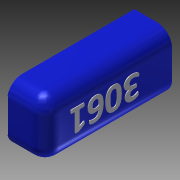
# Autodesk Inventor part: Bumper Cover Part4 (26x28 robot)
Saved by Autodesk Inventor 2014 SP1 (Build 180222100, 222)
## iProperties
Created: 2013-01-06
Part Number: Bumper Cover Part4 (26x28 robot)
Material: Generic
Document SubType Name: Modeling
Designer: Moses
Density: 1 g/cm^3
Mass: 183.688 g
Surface Area: 2193.04 cm^2
Volume: 183.688 cm^3
Appearance: Blue - Wall Paint - Glossy
Author: Moses
Autodesk Inventor part; units mm, degrees
ref_plane "YZ Plane" through (0, 0, 0) normal (1, 0, 0) x (0, 1, 0)
ref_plane "XZ Plane" through (0, 0, 0) normal (0, 1, 0) x (-1, 0, 0)
ref_plane "XY Plane" through (0, 0, 0) normal (0, 0, 1) x (1, 0, 0)
sketch "Sketch1" plane through (0, 0, 0) normal (0, 0, 1) x (1, 0, 0)
  circle A0 centre (38.1, -31.75) radius 31.75 construction
  circle A1 centre (38.1, 31.75) radius 31.75 construction
  line L0 (6.35, 63.5) -> (38.1, 63.5) construction
  line L1 (69.85, 31.75) -> (69.85, -31.75) construction
  line L2 (6.35, -63.5) -> (38.1, -63.5) construction
  line L3 (38.1, 65.0875) -> (-14.2875, 65.0875)
  line L4 (-14.2875, -65.0875) -> (38.1, -65.0875)
  arc A2 (38.1, -65.0875) -> (71.4375, -31.75) centre (38.1, -31.75) ccw
  arc A3 (71.4375, 31.75) -> (38.1, 65.0875) centre (38.1, 31.75) ccw
  line L5 (71.4375, 31.75) -> (71.4375, -31.75)
  line L6 (38.1, 65.0875) -> (38.1, 63.5) construction
  arc A4 (69.85, 31.75) -> (38.1, 63.5) centre (38.1, 31.75) ccw
  arc A5 (38.1, -63.5) -> (69.85, -31.75) centre (38.1, -31.75) ccw
  line L7 (69.85, 31.75) -> (69.85, -31.75)
  line L8 (-12.7, 63.5) -> (-12.7, 38.1)
  line L9 (-12.7, 38.1) -> (-14.2875, 38.1)
  line L10 (-14.2875, 38.1) -> (-14.2875, 65.0875)
  line L11 (-14.2875, -65.0875) -> (-14.2875, -38.1)
  line L12 (-14.2875, -38.1) -> (-12.7, -38.1)
  line L13 (-12.7, -63.5) -> (-12.7, -38.1)
  line L14 (-12.7, 38.1) -> (-12.7, -38.1)
  line L15 (-12.7, -63.5) -> (-12.7, 63.5) construction
  line L16 (-12.7, 63.5) -> (6.35, 63.5) construction
  line L17 (6.35, 63.5) -> (6.35, -63.5) construction
  line L18 (6.35, -63.5) -> (-12.7, -63.5) construction
  line L19 (-12.7, 63.5) -> (38.1, 63.5)
  line L20 (-12.7, -63.5) -> (38.1, -63.5)
  point P0 (0, 0)
  point P1 (38.1, 64.2937)
  dimension "d3" = 25.4
  dimension "d7" = 25.4
  dimension "d9" = 1.5875
  dimension "d20" = 1.5875
  dimension "d21" = 1.5875
  constraints: 34 end point, 14 tangent, 12 point on circle, 5 parallel, 4 centre point, 4 perpendicular, 2 coincident, 2 point on line, 1 collinear, 1 concentric, 1 midpoint, 1 vertical
  measures "d3" distance of L8.start L8.end
  measures "d7" distance of L13.start L12.end
  measures "d9" distance of L3.start L0.end
  measures "d20" distance of L11.end L12.end
  measures "d21" distance of L8.end L9.end
extrude "Extrusion1" add sketch "Sketch1" along normal blind 1.5875
extrude "Extrusion2" add sketch "Sketch1" against normal blind 285.75 contours A3 L5 A2 L4 L11 L12 L13 L20 A5 L7 A4 L19 L8 L9 L10 L3
sketch "Sketch2" plane through (0, 0, -285.75) normal (0, 0, -1) x (-1, 0, 0)
  arc A0 (-38.1, 63.5) -> (-69.85, 31.75) centre (-38.1, 31.75) ccw projected
  line L0 (-38.1, 63.5) -> (12.7, 63.5) projected
  line L1 (12.7, 63.5) -> (12.7, 38.1) projected
  line L2 (12.7, 38.1) -> (14.2875, 38.1) projected
  line L3 (14.2875, 38.1) -> (14.2875, 65.0875) projected
  line L4 (14.2875, 65.0875) -> (-38.1, 65.0875) projected
  arc A1 (-38.1, 65.0875) -> (-71.4375, 31.75) centre (-38.1, 31.75) ccw projected
  line L5 (-71.4375, 31.75) -> (-71.4375, -31.75) projected
  arc A2 (-71.4375, -31.75) -> (-38.1, -65.0875) centre (-38.1, -31.75) ccw projected
  line L6 (-38.1, -65.0875) -> (14.2875, -65.0875) projected
  line L7 (14.2875, -65.0875) -> (14.2875, -38.1) projected
  line L8 (14.2875, -38.1) -> (12.7, -38.1) projected
  line L9 (12.7, -38.1) -> (12.7, -63.5) projected
  line L10 (12.7, -63.5) -> (-38.1, -63.5) projected
  arc A3 (-69.85, -31.75) -> (-38.1, -63.5) centre (-38.1, -31.75) ccw projected
  line L11 (-69.85, -31.75) -> (-69.85, 31.75) projected
  line L12 (12.7, -63.5) -> (12.7, 63.5) projected
extrude "Extrusion3" add sketch "Sketch2" along normal blind 1.5875
fillet "Fillet1" radius 33.3375 8 edges at (61.6732, -55.3232, 1.5875) (71.4375, 0, 1.5875) (61.6732, 55.3232, 1.5875) (11.9063, 65.0875, 1.5875) (11.9062, -65.0875, 1.5875) (60.5506, -54.2006, 0) (69.85, 0, 0) (60.5506, 54.2006, 0)
sketch "Sketch3" plane through (71.4375, -31.75, -287.3375) normal (1, 0, 0) x (0, 0, -1)
  line L0 (-255.5875, 0) -> (-255.5875, 63.5) projected
  line L1 (0, 0) -> (-255.5875, 0) projected
  line L2 (0, 63.5) -> (-255.5875, 63.5) projected
  line L3 (-77.7875, 0) -> (-230.1875, 0) construction
  line L4 (-230.1875, 0) -> (-230.1875, 63.5) construction
  line L5 (-230.1875, 63.5) -> (-77.7875, 63.5) construction
  line L6 (-77.7875, 63.5) -> (-77.7875, 0) construction
  spline S0 degree 2 poles (-110.0562, 42.2439) (-110.0562, 46.0122) (-107.1466, 51.8792) (-101.995, 55.886) (-94.7924, 57.937) (-90.5471, 57.937) knots 0 0 0 1 2 3 4 4 4
  spline S1 degree 2 poles (-90.5471, 57.937) (-87.9714, 57.937) (-83.4399, 57.1738) (-79.9578, 56.1245) (-77.6683, 54.932) (-77.0005, 54.3119) (-76.6189, 53.501) (-76.3327, 52.4516) (-76.2373, 50.8775) (-76.2373, 49.7327) knots 0 0 0 1 2 3 4 5 6 7 8 8 8
  spline S2 degree 2 poles (-76.2373, 49.7327) (-76.2373, 47.8247) (-76.8574, 46.3938) (-77.4775, 46.3938) knots 0 0 0 1 2 2 2
  spline S3 degree 2 poles (-77.4775, 46.3938) (-77.8591, 46.3938) (-79.8147, 47.4431) (-82.7721, 48.6833) (-86.7789, 49.7327) (-89.3069, 49.7327) knots 0 0 0 1 2 3 4 4 4
  spline S4 degree 2 poles (-89.3069, 49.7327) (-91.4534, 49.7327) (-94.7447, 48.731) (-97.0343, 46.8707) (-98.179, 44.2473) (-98.179, 42.6732) knots 0 0 0 1 2 3 4 4 4
  spline S5 degree 2 poles (-98.179, 42.6732) (-98.179, 40.9083) (-96.7958, 38.094) (-94.1246, 36.0907) (-90.0224, 34.9936) (-87.2082, 34.9936) knots 0 0 0 1 2 3 4 4 4
  line L7 (-87.2082, 34.9936) -> (-82.8198, 34.9936)
  spline S6 degree 2 poles (-82.8198, 34.9936) (-82.3428, 34.9936) (-81.6273, 34.7074) (-81.1503, 33.8488) (-80.9595, 32.3224) (-80.9595, 31.1299) knots 0 0 0 1 2 3 4 4 4
  spline S7 degree 2 poles (-80.9595, 31.1299) (-80.9595, 29.9851) (-81.1503, 28.5541) (-81.5796, 27.7909) (-82.2474, 27.457) (-82.7244, 27.457) knots 0 0 0 1 2 3 4 4 4
  line L8 (-82.7244, 27.457) -> (-87.1605, 27.457)
  spline S8 degree 2 poles (-87.1605, 27.457) (-89.45, 27.457) (-92.9798, 26.4077) (-95.3648, 24.452) (-96.605, 21.6854) (-96.605, 19.9682) knots 0 0 0 1 2 3 4 4 4
  spline S9 degree 2 poles (-96.605, 19.9682) (-96.605, 18.6803) (-95.7464, 16.3908) (-94.0769, 14.7213) (-91.4057, 13.7196) (-89.5931, 13.7196) knots 0 0 0 1 2 3 4 4 4
  spline S10 degree 2 poles (-89.5931, 13.7196) (-87.5421, 13.7196) (-83.9646, 14.9121) (-81.1026, 16.3908) (-79.0992, 17.6309) (-78.6222, 17.6309) knots 0 0 0 1 2 3 4 4 4
  spline S11 degree 2 poles (-78.6222, 17.6309) (-78.336, 17.6309) (-77.8591, 17.3447) (-77.5252, 16.5815) (-77.3821, 15.1029) (-77.3821, 13.9104) knots 0 0 0 1 2 3 4 4 4
  spline S12 degree 2 poles (-77.3821, 13.9104) (-77.3821, 12.9564) (-77.4775, 11.6685) (-77.716, 10.8099) (-78.0498, 10.1898) (-78.813, 9.4266) (-81.2457, 7.9479) (-84.9186, 6.5169) (-89.7362, 5.563) (-92.5505, 5.563) knots 0 0 0 1 2 3 4 5 6 7 8 8 8
  spline S13 degree 2 poles (-92.5505, 5.563) (-96.2234, 5.563) (-101.8996, 7.2801) (-105.7633, 10.5237) (-107.7667, 15.246) (-107.7667, 18.251) knots 0 0 0 1 2 3 4 4 4
  spline S14 degree 2 poles (-107.7667, 18.251) (-107.7667, 20.5406) (-106.5742, 24.4997) (-104.3323, 27.6478) (-100.8979, 29.842) (-98.7037, 30.3667) knots 0 0 0 1 2 3 4 4 4
  line L9 (-98.7037, 30.3667) -> (-98.7037, 30.5098)
  spline S15 degree 2 poles (-98.7037, 30.5098) (-101.3272, 30.796) (-105.5725, 32.8948) (-108.4821, 35.9953) (-110.0562, 39.9543) (-110.0562, 42.2439) knots 0 0 0 1 2 3 4 4 4
  spline S16 degree 2 poles (-151.841, 31.5592) (-151.841, 37.617) (-149.8853, 47.3954) (-145.4493, 54.2642) (-138.3898, 57.937) (-133.2859, 57.937) knots 0 0 0 1 2 3 4 4 4
  spline S17 degree 2 poles (-133.2859, 57.937) (-128.0867, 57.937) (-121.2656, 54.3596) (-117.3066, 47.6816) (-115.6848, 38.0463) (-115.6848, 31.9408) knots 0 0 0 1 2 3 4 4 4
  spline S18 degree 2 poles (-115.6848, 31.9408) (-115.6848, 25.9307) (-117.6882, 16.1046) (-122.0765, 9.2358) (-129.1837, 5.563) (-134.2399, 5.563) knots 0 0 0 1 2 3 4 4 4
  spline S19 degree 2 poles (-134.2399, 5.563) (-139.4391, 5.563) (-146.3079, 9.1404) (-150.2669, 15.8184) (-151.841, 25.4537) (-151.841, 31.5592) knots 0 0 0 1 2 3 4 4 4
  spline S20 degree 2 poles (-141.4902, 32.0362) (-141.4902, 28.4587) (-141.1086, 22.9256) (-140.2977, 18.8711) (-139.0575, 16.0569) (-137.3404, 14.3874) (-135.1462, 13.6719) (-133.8106, 13.6719) knots 0 0 0 1 2 3 4 5 6 6 6
  spline S21 degree 2 poles (-133.8106, 13.6719) (-131.521, 13.6719) (-128.516, 15.9138) (-126.7511, 20.3498) (-126.0356, 27.0277) (-126.0356, 31.4161) knots 0 0 0 1 2 3 4 4 4
  spline S22 degree 2 poles (-126.0356, 31.4161) (-126.0356, 36.8538) (-126.8942, 43.9134) (-128.7544, 48.1109) (-131.6164, 49.7804) (-133.6675, 49.7804) knots 0 0 0 1 2 3 4 4 4
  spline S23 degree 2 poles (-133.6675, 49.7804) (-135.1939, 49.7804) (-137.5312, 48.7787) (-139.296, 46.8231) (-140.4885, 43.8657) (-141.204, 39.9543) (-141.4902, 35.0413) (-141.4902, 32.0362) knots 0 0 0 1 2 3 4 5 6 6 6
  spline S24 degree 2 poles (-192.1471, 40.1451) (-192.1471, 43.9611) (-189.8098, 50.4959) (-185.2784, 55.2182) (-178.6005, 57.937) (-174.2598, 57.937) knots 0 0 0 1 2 3 4 4 4
  spline S25 degree 2 poles (-174.2598, 57.937) (-170.7777, 57.937) (-165.5308, 56.3153) (-161.7148, 53.3102) (-159.2821, 49.0172) (-157.8035, 43.6272) (-157.2788, 37.2831) (-157.2788, 33.7534) knots 0 0 0 1 2 3 4 5 6 6 6
  spline S26 degree 2 poles (-157.2788, 33.7534) (-157.2788, 30.796) (-157.8512, 24.3089) (-159.5683, 18.0602) (-162.6211, 12.384) (-167.3911, 8.091) (-174.2598, 5.6107) (-178.9344, 5.6107) knots 0 0 0 1 2 3 4 5 6 6 6
  spline S27 degree 2 poles (-178.9344, 5.6107) (-180.413, 5.6107) (-183.4658, 5.9446) (-186.0416, 6.5169) (-187.8065, 7.2324) (-188.4266, 7.7094) (-188.7128, 8.3295) (-188.9036, 9.0927) (-188.999, 10.1898) (-188.999, 10.953) knots 0 0 0 1 2 3 4 5 6 7 8 8 8
  spline S28 degree 2 poles (-188.999, 10.953) (-188.999, 12.1932) (-188.9036, 13.815) (-188.5697, 14.6736) (-187.9973, 15.1029) (-187.6157, 15.1029) knots 0 0 0 1 2 3 4 4 4
  spline S29 degree 2 poles (-187.6157, 15.1029) (-187.1387, 15.1029) (-185.66, 14.5782) (-183.5612, 13.9581) (-180.6992, 13.4811) (-178.839, 13.4811) knots 0 0 0 1 2 3 4 4 4
  spline S30 degree 2 poles (-178.839, 13.4811) (-175.6431, 13.4811) (-171.2547, 15.8184) (-168.5359, 19.8251) (-167.2957, 25.1198) (-167.248, 28.0771) knots 0 0 0 1 2 3 4 4 4
  spline S31 degree 2 poles (-167.248, 28.0771) (-168.1066, 27.5524) (-170.3484, 26.4554) (-172.9719, 25.6922) (-175.977, 25.1675) (-177.7419, 25.1675) knots 0 0 0 1 2 3 4 4 4
  spline S32 degree 2 poles (-177.7419, 25.1675) (-181.5578, 25.1675) (-187.0433, 27.2662) (-190.5253, 31.1776) (-192.1471, 36.7584) (-192.1471, 40.1451) knots 0 0 0 1 2 3 4 4 4
  spline S33 degree 2 poles (-182.0825, 41.0991) (-182.0825, 39.1434) (-181.367, 36.0907) (-179.7929, 34.0396) (-177.2172, 32.9902) (-175.4046, 32.9902) knots 0 0 0 1 2 3 4 4 4
  spline S34 degree 2 poles (-175.4046, 32.9902) (-174.3075, 32.9902) (-172.161, 33.3718) (-170.1576, 34.0873) (-168.2497, 35.0413) (-167.4388, 35.6137) knots 0 0 0 1 2 3 4 4 4
  spline S35 degree 2 poles (-167.4388, 35.6137) (-167.4388, 39.7635) (-168.3928, 45.3921) (-170.2053, 48.6356) (-173.0196, 50.0189) (-174.8322, 50.0189) knots 0 0 0 1 2 3 4 4 4
  spline S36 degree 2 poles (-174.8322, 50.0189) (-176.6448, 50.0189) (-179.3636, 48.6833) (-181.1285, 46.2507) (-182.0825, 43.0071) (-182.0825, 41.0991) knots 0 0 0 1 2 3 4 4 4
  spline S37 degree 2 poles (-231.4515, 53.1194) (-231.4515, 54.2165) (-231.213, 55.7429) (-230.7837, 56.6492) (-230.259, 57.0307) (-229.8775, 57.0307) knots 0 0 0 1 2 3 4 4 4
  line L10 (-229.8775, 57.0307) -> (-201.9732, 57.0307)
  spline S38 degree 2 poles (-201.9732, 57.0307) (-201.6393, 57.0307) (-201.1146, 56.6492) (-200.6853, 55.7429) (-200.4468, 54.2165) (-200.4468, 53.1194) knots 0 0 0 1 2 3 4 4 4
  spline S39 degree 2 poles (-200.4468, 53.1194) (-200.4468, 52.0223) (-200.6376, 50.4959) (-201.0669, 49.5419) (-201.6393, 49.1126) (-201.9732, 49.1126) knots 0 0 0 1 2 3 4 4 4
  line L11 (-201.9732, 49.1126) -> (-211.37, 49.1126)
  line L12 (-211.37, 49.1126) -> (-211.37, 16.1523)
  line L13 (-211.37, 16.1523) -> (-203.2134, 20.636)
  spline S40 degree 2 poles (-203.2134, 20.636) (-202.3548, 21.0653) (-201.21, 21.2561) (-200.5422, 20.5883) (-200.3037, 18.9665) (-200.3037, 17.4878) knots 0 0 0 1 2 3 4 4 4
  spline S41 degree 2 poles (-200.3037, 17.4878) (-200.3037, 16.5338) (-200.3991, 15.3414) (-200.6853, 14.4828) (-201.2577, 13.9104) (-201.7347, 13.6242) knots 0 0 0 1 2 3 4 4 4
  line L14 (-201.7347, 13.6242) -> (-212.5625, 6.6123)
  spline S42 degree 2 poles (-212.5625, 6.6123) (-212.801, 6.4215) (-213.3734, 6.2308) (-214.3274, 6.1354) (-215.8538, 6.0877) (-217.0463, 6.0877) knots 0 0 0 1 2 3 4 4 4
  spline S43 degree 2 poles (-217.0463, 6.0877) (-218.525, 6.0877) (-220.3852, 6.1831) (-221.2915, 6.4692) (-221.6254, 6.9462) (-221.6254, 7.2801) knots 0 0 0 1 2 3 4 4 4
  line L15 (-221.6254, 7.2801) -> (-221.6254, 49.1126)
  line L16 (-221.6254, 49.1126) -> (-229.8775, 49.1126)
  spline S44 degree 2 poles (-229.8775, 49.1126) (-230.259, 49.1126) (-230.8314, 49.5419) (-231.2607, 50.4959) (-231.4515, 52.0223) (-231.4515, 53.1194) knots 0 0 0 1 2 3 4 4 4
  point P0 (-287.3375, 31.75)
  point P1 (-1.5875, 0)
  point P2 (-1.5875, 63.5)
  dimension "d0" = 1.5875
  dimension "d1" = 0
  dimension "d15" = 152.4
  dimension "d17" = 25.4
  constraints: 2 point on line, 2 other
  measures "d15" distance of L3.start L3.end
  measures "d17" distance between parallel lines of L0 L4
extrude "Extrusion4" add sketch "Sketch3" along normal blind 1.5875
body "Solid1"
